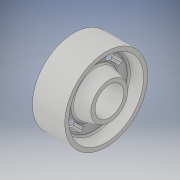
# Autodesk Inventor part: koło_zapasowe
Saved by Autodesk Inventor 2019 (Build 230136000, 136)
## iProperties
Created: 2019-05-26
Part Number: koło_zapasowe
Material: Ogólny
Document SubType Name: Modeling
Designer: student
Density: 1 g/cm^3
Appearance: Domyślna
Author: student
Autodesk Inventor part; units mm, degrees
ref_plane "YZ Plane" through (0, 0, 0) normal (1, 0, 0) x (0, 1, 0)
ref_plane "XZ Plane" through (0, 0, 0) normal (0, 1, 0) x (-1, 0, 0)
ref_plane "XY Plane" through (0, 0, 0) normal (0, 0, 1) x (1, 0, 0)
sketch "Szkic1" plane through (0, 0, 0) normal (0, 0, 1) x (1, 0, 0)
  line L0 (18, 25.5) -> (30.0527, 25.5) construction
  line L1 (21.5, 0) -> (21.5, 4.5)
  line L2 (21.5, 4.5) -> (6.358, 8.5573)
  line L3 (4.8757, 10.4891) -> (4.8757, 20.4487)
  line L4 (0, 0) -> (21.5, 0)
  line L5 (-18, 30) -> (-18, 25.5)
  line L6 (-18, 25.5) -> (-6.358, 22.3805)
  line L7 (0, 0) -> (-21.5, 0)
  line L8 (-4.8757, 10.4891) -> (-4.8757, 20.4487)
  arc A0 (-4.8757, 20.4487) -> (-6.358, 22.3805) centre (-6.8757, 20.4487) ccw
  arc A1 (-6.358, 8.5573) -> (-4.8757, 10.4891) centre (-6.8757, 10.4891) ccw
  arc A2 (6.358, 22.3805) -> (4.8757, 20.4487) centre (6.8757, 20.4487) ccw
  arc A3 (4.8757, 10.4891) -> (6.358, 8.5573) centre (6.8757, 10.4891) ccw
  line L9 (-6.358, 8.5573) -> (-21.5, 4.5)
  line L10 (21.5, 4.5) -> (6.358, 8.5573)
  line L11 (6.358, 22.3805) -> (18, 25.5)
  line L12 (18, 30) -> (18, 25.5)
  line L13 (0, 30) -> (-18, 30)
  line L14 (-21.5, 4.5) -> (-21.5, 0)
  line L15 (18, 30) -> (-18, 30)
  line L16 (21.5, -16) -> (-21.5, -16)
  point P0 (-4.8757, 21.9833)
  point P1 (-4.8757, 8.9545)
  dimension "d0" = 30
  dimension "d1" = 18
  dimension "d2" = 4.5
  dimension "d4" = 21.5
  dimension "d5" = 4.5
  dimension "d6" = 105
  dimension "d7" = 2
  dimension "d13" = 43
  constraints: 34 end point, 8 point on circle, 4 centre point, 3 point on line, 1 horizontal
  measures "d0" distance of L4.start L13.start
  measures "d1" distance of L13.start L12.start
  measures "d2" distance of L12.start L0.start
  measures "d4" distance of L4.start L1.start
  measures "d5" distance of L1.start L1.end
  measures "d6" angle of L2 L1
  measures "d7" radius of A0
  measures "d13" distance of L16.start L16.end
revolve "Obrót1" add sketch "Szkic1" angle 360 about axis through (21.5, -16, 0) along (-1, 0, 0)
sketch "Szkic2" plane through (4.8757, -16, 0) normal (1, 0, 0) x (0, 0, -1)
  circle A0 centre (0, 0) radius 35 construction
  circle A1 centre (0, 0) radius 28 construction
  line L0 (0, 0) -> (23.915, 51.2858) construction
  line L1 (0, 0) -> (56.5876, 0) construction
  line L2 (0, 0) -> (50.5859, 23.5886) construction
  line L3 (0, 0) -> (55.8154, 0) construction
  line L4 (13.9208, 29.8532) -> (12.7771, 27.4006)
  line L5 (27.1158, 12.6443) -> (29.8532, 13.9208)
  arc A2 (30.766, 16.6869) -> (16.6869, 30.766) centre (0, 0) ccw
  arc A3 (16.6869, 30.766) -> (13.9208, 29.8532) centre (15.7334, 29.0079) ccw
  arc A4 (29.8532, 13.9208) -> (30.766, 16.6869) centre (29.0079, 15.7334) ccw
  arc A5 (24.4846, 13.5569) -> (27.1158, 12.6443) centre (26.2706, 14.4569) ccw
  line L6 (12.7771, 27.4006) -> (12.6503, 27.1287)
  arc A6 (12.6503, 27.1287) -> (13.4988, 24.5313) centre (14.463, 26.2835) ccw
  arc A7 (24.4846, 13.5569) -> (13.4988, 24.5313) centre (0.1262, 0.159) ccw
  arc A8 (-16.4016, 30.7988) -> (-30.4807, 16.7197) centre (0.2853, 0.0328) ccw
  line L7 (-29.5679, 13.9536) -> (-26.8435, 12.6831)
  arc A9 (-26.8435, 12.6831) -> (-24.246, 13.5316) centre (-25.9982, 14.4958) ccw
  arc A10 (-13.2716, 24.5174) -> (-24.246, 13.5316) centre (0.1262, 0.159) ccw
  arc A11 (-13.2716, 24.5174) -> (-12.359, 27.1486) centre (-14.1717, 26.3034) ccw
  arc A12 (-30.4807, 16.7197) -> (-29.5679, 13.9536) centre (-28.7227, 15.7662) ccw
  arc A13 (-13.6355, 29.886) -> (-16.4016, 30.7988) centre (-15.4481, 29.0407) ccw
  line L8 (-12.359, 27.1486) -> (-13.6355, 29.886)
  arc A14 (-30.5135, -16.3688) -> (-16.4344, -30.4479) centre (0.2525, 0.3181) ccw
  line L9 (-13.6683, -29.5351) -> (-12.3979, -26.8107)
  arc A15 (-12.3979, -26.8107) -> (-13.2463, -24.2132) centre (-14.2105, -25.9654) ccw
  arc A16 (-24.2321, -13.2388) -> (-13.2463, -24.2132) centre (0.1262, 0.159) ccw
  arc A17 (-24.2321, -13.2388) -> (-26.8634, -12.3263) centre (-26.0181, -14.1389) ccw
  arc A18 (-16.4344, -30.4479) -> (-13.6683, -29.5351) centre (-15.4809, -28.6899) ccw
  arc A19 (-29.6007, -13.6027) -> (-30.5135, -16.3688) centre (-28.7555, -15.4153) ccw
  line L10 (-26.8634, -12.3263) -> (-29.6007, -13.6027)
  arc A20 (16.6541, -30.4807) -> (30.7332, -16.4016) centre (-0.0328, 0.2853) ccw
  line L11 (29.8204, -13.6355) -> (27.0959, -12.3651)
  arc A21 (27.0959, -12.3651) -> (24.4985, -13.2135) centre (26.2507, -14.1777) ccw
  arc A22 (13.5241, -24.1993) -> (24.4985, -13.2135) centre (0.1262, 0.159) ccw
  arc A23 (13.5241, -24.1993) -> (12.6115, -26.8306) centre (14.4241, -25.9853) ccw
  arc A24 (30.7332, -16.4016) -> (29.8204, -13.6355) centre (28.9751, -15.4481) ccw
  arc A25 (13.888, -29.5679) -> (16.6541, -30.4807) centre (15.7006, -28.7227) ccw
  line L12 (12.6115, -26.8306) -> (13.888, -29.5679)
  point P0 (0, 16)
  point P1 (14.7916, 31.7208)
  point P2 (25.293, 11.7943)
  point P3 (31.7208, 14.7916)
  point P4 (11.8333, 25.3766)
  dimension "d16" = 56
  dimension "d15" = 70
  dimension "d17" = 65
  dimension "d18" = 25
  dimension "d19" = 2
  dimension "d21" = 2
  dimension "d22" = 2
  constraints: 52 point on circle, 26 end point, 25 centre point, 7 point on line, 6 tangent, 2 coincident, 2 equal length, 2 equal radius, 2 horizontal, 1 collinear, 1 midpoint, 3 other
  measures "d15" diameter of A0
  measures "d17" angle of L1 L0
  measures "d18" angle of L3 L2
  measures "d19" radius of A3
  measures "d21" radius of A4
  measures "d22" radius of A6
extrude "Wyciągnięcie proste1" cut sketch "Szkic2" against normal blind 30 and the other way blind 15
